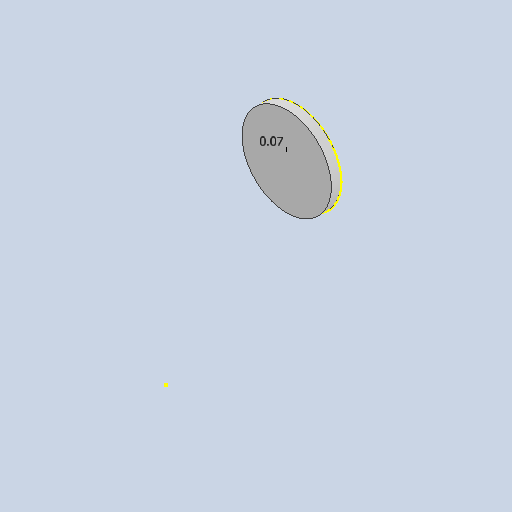
# Autodesk Inventor part: pinEndCap_V3
Saved by Autodesk Inventor 2023 (Build 270158000, 158)
## iProperties
Created: 2022-11-25
Part Number: pinEndCap_V3
Material: Generic
Document SubType Name: Modeling
Designer: shrey
Density: 1 g/cm^3
Appearance: Default
Author: shrey
Autodesk Inventor part; units mm, degrees
ref_plane "YZ Plane" through (0, 0, 0) normal (1, 0, 0) x (0, 1, 0)
ref_plane "XZ Plane" through (0, 0, 0) normal (0, 1, 0) x (-1, 0, 0)
ref_plane "XY Plane" through (0, 0, 0) normal (0, 0, 1) x (1, 0, 0)
ref_plane "Work Plane1" through (26.746, 54.122, -10.1057) normal (0, 0, 1) x (1, 0, 0)
sketch "Sketch1" plane through (26.746, 54.122, -10.1057) normal (0, 0, 1) x (1, 0, 0)
  circle A0 centre (0, 0) radius 3.86 construction
  circle A1 centre (0, 0) radius 3.79
  circle A2 centre (0, 0) radius 9.16 projected
  point P0 (-26.746, -54.122)
  dimension "d0" = 0.07
  constraints: 1 centre point
  measures "d0" radial gap between concentric circles of A0 A1
extrude "Extrusion1" add sketch "Sketch1" along normal blind 2 contours A1 | A2
extrude "Extrusion2" add sketch "Sketch1" against normal blind 3 contours A1
body "Solid1"
